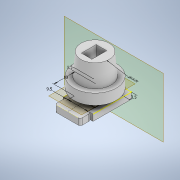
# Autodesk Inventor part: Ant connector
Saved by Autodesk Inventor 2022 (Build 260153070, 153G)
## iProperties
Created: 2021-09-17
Part Number: Ant connector
Material: Generic
Document SubType Name: Modeling
Designer: cb2409
Density: 1 g/cm^3
Appearance: Default
Author: cb2409
Autodesk Inventor part; units mm, degrees
ref_plane "YZ Plane" through (0, 0, 0) normal (1, 0, 0) x (0, 1, 0)
ref_plane "XZ Plane" through (0, 0, 0) normal (0, 1, 0) x (-1, 0, 0)
ref_plane "XY Plane" through (0, 0, 0) normal (0, 0, 1) x (1, 0, 0)
sketch "Sketch3" plane through (0, 0, 0) normal (0, 1, 0) x (-1, 0, 0)
  spline S0 degree 3 poles (2.0049, 23.0048) (1.4509, 23.0048) (1.005, 22.5589) (1.005, 22.0049) knots 0 0 0 0 1 1 1 1
  line L0 (2.0049, 23.0048) -> (1.4509, 23.0048) construction
  line L1 (1.4509, 23.0048) -> (1.005, 22.5589) construction
  line L2 (1.005, 22.5589) -> (1.005, 22.0049) construction
  spline S1 degree 3 poles (1.005, 19.0051) (1.005, 18.4511) (1.4509, 18.0046) (2.0049, 18.0046) knots 0 0 0 0 1 1 1 1
  line L3 (1.005, 19.0051) -> (1.005, 18.4511) construction
  line L4 (1.005, 18.4511) -> (1.4509, 18.0046) construction
  line L5 (1.4509, 18.0046) -> (2.0049, 18.0046) construction
  line L6 (1.005, 22.0049) -> (1.005, 19.0051)
  spline S2 degree 3 poles (12.0053, 18.0046) (12.5593, 18.0046) (13.0053, 18.4511) (13.0053, 19.0051) knots 0 0 0 0 1 1 1 1
  line L7 (12.0053, 18.0046) -> (12.5593, 18.0046) construction
  line L8 (12.5593, 18.0046) -> (13.0053, 18.4511) construction
  line L9 (13.0053, 18.4511) -> (13.0053, 19.0051) construction
  line L10 (2.0049, 18.0046) -> (0.005, 18.0046)
  line L11 (0.005, 18.0046) -> (0.005, 0.0047)
  line L12 (0.005, 0.0047) -> (14.0052, 0.0048)
  line L13 (14.0052, 0.0048) -> (14.0052, 18.0046)
  line L14 (14.0052, 18.0046) -> (12.0053, 18.0046)
  spline S3 degree 3 poles (13.0053, 22.0049) (13.0053, 22.5589) (12.5593, 23.0048) (12.0053, 23.0048) knots 0 0 0 0 1 1 1 1
  line L15 (13.0053, 22.0049) -> (13.0053, 22.5589) construction
  line L16 (13.0053, 22.5589) -> (12.5593, 23.0048) construction
  line L17 (12.5593, 23.0048) -> (12.0053, 23.0048) construction
  line L18 (13.0053, 19.0051) -> (13.0053, 22.0049)
  line L19 (12.0053, 23.0048) -> (2.0049, 23.0048)
  point P0 (0, 0)
  point P1 (2.0049, 23.0048)
  point P2 (1.005, 22.0049)
  point P3 (1.005, 19.0051)
  point P4 (2.0049, 18.0046)
  point P5 (0.005, 18.0046)
  point P6 (12.0054, 18.0046)
  point P7 (12.0053, 23.0048)
  constraints: 16 end point, 12 other
extrude "Extrusion2" add sketch "Sketch3" along normal blind 3
ref_plane "Edge of module" through (0, 6.1, 0) normal (0, 1, 0) x (1, 0, 0)
sketch "Sketch5" plane through (0, 3, 0) normal (0, 1, 0) x (1, 0, 0)
  line L0 (-0.005, -18.0046) -> (-0.005, -0.0047) projected
  line L1 (-0.005, -3.5047) -> (-14.0052, -3.5048) construction
  line L2 (-14.0052, -0.0048) -> (-14.0052, -18.0046) projected
  line L3 (-0.005, -0.0047) -> (-14.0052, -0.0048) projected
  line L4 (-0.005, -0.0047) -> (-14.0052, -0.0048) construction
  line L5 (-7.0051, -0.0047) -> (-7.0051, -23.0048) construction
  line L6 (-12.0053, -23.0048) -> (-2.0049, -23.0048) construction
  line L7 (-2.2551, -15.0047) -> (-2.2551, -5.0047)
  line L8 (-2.2551, -5.0047) -> (-11.7551, -5.0047)
  line L9 (-11.7551, -5.0047) -> (-11.7551, -15.0047)
  line L10 (-11.7551, -15.0047) -> (-2.2551, -15.0047)
  line L11 (-2.2551, -15.0047) -> (-11.7551, -5.0047) construction
  line L12 (-2.2551, -5.0047) -> (-11.7551, -15.0047) construction
  point P0 (0, 0)
  point P1 (-7.0051, -10.0047)
  dimension "d9" = 3.5
  dimension "d10" = 9.5
  dimension "d11" = 10
  dimension "d12" = 1.5
  constraints: 16 end point, 4 midpoint, 3 parallel, 3 point on line, 1 perpendicular
  measures "d9" distance between parallel lines of L3 L1
  measures "d10" distance of L9.end L7.start
  measures "d11" distance of L8.end L9.end
  measures "d12" distance between parallel lines of L8 L1
extrude "Extrusion3" add sketch "Sketch5" along normal up to surface (3.1 mm away)
sketch "Sketch6" plane through (-11.7551, 6.1, 5.0047) normal (0, 1, 0) x (1, 0, 0)
  line L0 (4.75, 5) -> (4.75, -18.0001) construction
  line L1 (9.5, -10) -> (0, -10) construction
  line L2 (9.5, -10) -> (0, 0) construction
  circle A0 centre (4.75, -5) radius 10
  point P0 (11.7551, 5.0047)
  dimension "d15" = 20
  constraints: 2 end point, 1 centre point, 1 midpoint
  measures "d15" diameter of A0
extrude "Extrusion4" add sketch "Sketch6" along normal blind 5
sketch "Sketch7" plane through (-7.0051, 11.1, 10.0047) normal (0, 1, 0) x (1, 0, 0)
  circle A0 centre (0, 0) radius 7.5
  point P0 (7.0051, 10.0047)
  dimension "d18" = 15
  constraints: 1 centre point
  measures "d18" diameter of A0
extrude "Extrusion5" add sketch "Sketch7" along normal blind 10 draft -5
ref_plane "Work Plane5" through (-0.005, 0, 0.0047) normal (0, 0, -1) x (-1, 0, 0)
sketch "Sketch8" plane through (0, 0, 0) normal (0, -1, 0) x (1, 0, 0)
  line L0 (-9.5051, 7.0047) -> (-4.5051, 7.0047)
  line L1 (-4.5051, 7.0047) -> (-4.5051, 14.0047)
  line L2 (-4.5051, 14.0047) -> (-9.5051, 14.0047)
  line L3 (-9.5051, 14.0047) -> (-9.5051, 7.0047)
  line L4 (-9.5051, 7.0047) -> (-4.5051, 14.0047) construction
  line L5 (-4.5051, 7.0047) -> (-9.5051, 14.0047) construction
  line L6 (-0.005, 0.0047) -> (-14.0052, 0.0048) construction
  line L7 (-7.0051, 0.0047) -> (-7.0051, 22.9634) construction
  line L8 (2.801, 0.0047) -> (-16.8063, 0.0048) projected
  point P0 (0, 0)
  point P1 (-7.0051, 10.5047)
  dimension "d21" = 5
  dimension "d22" = 7
  dimension "d24" = 7
  constraints: 14 end point, 3 midpoint, 2 parallel, 1 horizontal, 1 perpendicular, 1 point on line, 1 vertical
  measures "d21" distance of L1.end L2.end
  measures "d22" distance of L0.end L1.end
  measures "d24" distance from line of L8 L0.end
extrude "Extrusion6" cut sketch "Sketch8" against normal through all
body "Solid2"
